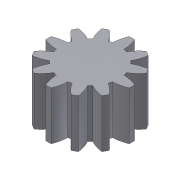
# Autodesk Inventor part: 12 Tooth Pinion Gear
Saved by Autodesk Inventor 2014 (Build 180170000, 170)
## iProperties
Created: 2007-12-06
Material: Steel
Document SubType Name: Modeling
Density: 7.85 g/cm^3
Mass: 28.0318 g
Surface Area: 20.5817 cm^2
Volume: 3.57093 cm^3
Project: FIRST
Description: 12 Tooth Pinion Gear for Keyang motor
Vendor: Keyang
Appearance: Steel
CustomPartVersion: 1
Category: Motors
Title: 12 Tooth Pinion Gear
Author: Autodesk, Inc.
Autodesk Inventor part; units mm, degrees
sketch "Sketch1" plane through (0, 0, 0) normal (0, 0, 1) x (1, 0, 0)
  circle A0 centre (0, 0) radius 11
  dimension "d0" = 22
  constraints: 1 centre point
  measures "d0" diameter of A0
extrude "Extrusion1" add sketch "Sketch1" along normal blind 12.75
ref_plane "Work Plane2" through (0, 0, 6.375) normal (0, 0, 1) x (1, 0, 0)
sketch "Sketch2" plane through (0, 0, 0) normal (0, 0, -1) x (-1, 0, 0)
  circle A0 centre (0, 0) radius 11 projected
  circle A1 centre (0, 0) radius 9.525
  dimension "d3" = 19.05
  constraints: 1 centre point, 1 coincident
  measures "d3" diameter of A1
surface extrude "ExtrusionSrf1" sketch "Sketch2" against normal through all shown no curves A1
ref_plane "Work Plane8" through (0, 0, 0) normal (0.9659258, 0.258819, 0) x (0, 0, 1)
ref_plane "Work Plane9" through (0, 0, 0) normal (1, 0, 0) x (0, 1, 0)
spur gear teeth "Spur Gear" teeth 12 pitch diameter 19.05 tip diameter 22 root diameter 15.081 face width 12.75 start plane through (0, 0, 0) normal (0, 0, -1) x (-1, 0, 0)
equation "\"d0\" = da_da"
equation "\"d1\" = da_b"
equation "\"d3\" = da_dw"
equation "\"d16\" = da_aw"
equation "\"d43\" = da_aw"
equation "\"d46\" = da_aw"
equation "\"da_da\" = 22"
equation "\"da_b\" = 12.75"
equation "\"da_dw\" = 19.05"
equation "\"da_aw\" = 19.05"
body "Solid1"
body "Srf1"
